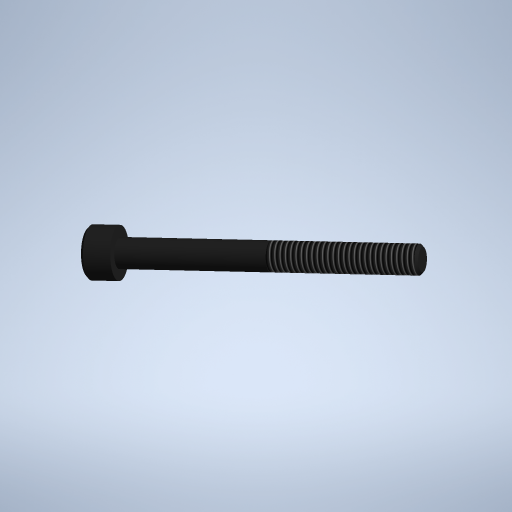
# Autodesk Inventor part: SCREW, SOCKET HD, P, 12.9, M4X0.7X40MM
Saved by Autodesk Inventor 2024.2 (Build 282272000, 272)
## iProperties
Category: _
Manager: 100-05647
Created: 2001-02-20
Part Number: SCREW, SOCKET HD, P, 12.9, M4X0.7X40MM
Material: Steel, MS
Document SubType Name: Modeling
Designer: cdotson
Density: 7.86 g/cm^3
Appearance: Black
Mfg Approved By: Clint.Matte
Mass: 5.01762 g
Surface Area: 6.79859 cm^2
Volume: 0.638374 cm^3
Checked By: 0002069160
User Status: Released
Description: SCREW, SOCKET HD, P, 12.9, M4X0.7X40MM
Engr Approved By: P
Control State: 0
Master: False
Checked Out: False
Shininess: 64.0
CN_MASS: 0.005018
FIRST_DESCRIPTION: SCREW, SOCKET HD, P, 12.9, M4X0.7X40MM
SECOND_DESCRIPTION: _
THIRD_DESCRIPTION: _
CN_SERVICEABLE: _
PTC_WM_ITERATION: 2
PTC_WM_ORGANIZATION_ID: CLWC
PTC_WM_LIFECYCLE: CLWC_CAD_LC
CL_runCount: 1
FinishProperty: ToBeSet
CN_MFG_PART_NUM: _
Density: 0.0
Volumn: 0.0
Area: 0.0
PropertySet Name: Model Information
Author: -
Revision Number: A
Keywords: DEFAULT
Subject: _
Autodesk Inventor part; units mm, degrees
ref_plane "YZ Plane" through (0, 0, 0) normal (1, 0, 0) x (0, 1, 0)
ref_plane "XZ Plane" through (0, 0, 0) normal (0, 1, 0) x (-1, 0, 0)
ref_plane "XY Plane" through (0, 0, 0) normal (0, 0, 1) x (1, 0, 0)
sketch "Sketch1" plane through (0, 0, 0) normal (0, 0, 1) x (1, 0, 0)
  circle A0 centre (0, 0) radius 2
  dimension "Diameter" = 4
  constraints: 1 centre point
  measures "Diameter" diameter of A0
extrude "Extrusion1" add sketch "Sketch1" along normal blind 40
sketch "Sketch2" plane through (0, 0, 40) normal (0, 0, 1) x (1, 0, 0)
  circle A0 centre (0, 0) radius 2 projected
  circle A1 centre (0, 0) radius 3.5
  dimension "Head_Diameter" = 7
  constraints: 1 centre point, 1 coincident
  measures "Head_Diameter" diameter of A1
extrude "Extrusion2" add sketch "Sketch2" along normal blind 4 contours A0 | A1
sketch "Sketch3" plane through (0, 0, 44) normal (0, 0, 1) x (1, 0, 0)
  circle A0 centre (0, 0) radius 3.5 projected
  circle A1 centre (0, 0) radius 1.7321 construction
  line L0 (0, 1.7321) -> (1.5, 0.866)
  line L1 (1.5, -0.866) -> (1.5, 0.866)
  line L2 (0, 1.7321) -> (-1.5, 0.866)
  line L3 (-1.5, -0.866) -> (-1.5, 0.866)
  line L4 (-1.5, -0.866) -> (0, -1.7321)
  line L5 (1.5, -0.866) -> (0, -1.7321)
  dimension "Hex_Width" = 3
  constraints: 12 end point, 6 point on circle, 3 equal length, 1 centre point, 1 coincident, 1 parallel, 1 vertical
  measures "Hex_Width" distance between parallel lines of L0 L4
extrude "Extrusion3" cut sketch "Sketch3" against normal blind 2 contours L0 L1 L5 L4 L3 L2
thread "Thread1" size "M4x0.7" class "4g6g" standard "ANSI Metric M Profile" length 20
chamfer "Chamfer1" distance 0.4 angle 45 2 edges at (-3.5, 0, 44) (-2, 0, 0)
equation "\"d9\" = ThreadLength"
equation "\"d12\" = Chamfer"
equation "\"ThreadLength\" = 20"
equation "\"Chamfer\" = 0.4"
body "Solid1"
